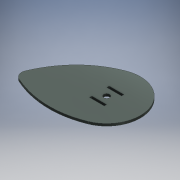
# Autodesk Inventor part: leva00
Saved by Autodesk Inventor 2016 (Build 200138000, 138)
## iProperties
Created: 2016-09-20
Part Number: leva00
Material: Madera (abedul)
Document SubType Name: Modeling
Designer: i95sa
Density: 0.55 g/cm^3
Appearance: Gris plomo - Pulido
Author: i95sa
Autodesk Inventor part; units mm, degrees
ref_plane "YZ Plane" through (0, 0, 0) normal (1, 0, 0) x (0, 1, 0)
ref_plane "XZ Plane" through (0, 0, 0) normal (0, 1, 0) x (-1, 0, 0)
ref_plane "XY Plane" through (0, 0, 0) normal (0, 0, 1) x (1, 0, 0)
sketch "Boceto1" plane through (0, 0, 0) normal (0, 0, 1) x (1, 0, 0)
  arc A0 (52.8206, 20.9132) -> (-52.8206, -20.9132) centre (0, 0) ccw
  arc A1 (-81.2867, -32.1837) -> (-105.6655, -41.8359) centre (-93.4761, -37.0098) ccw
  line L0 (-109.1946, -43.2332) -> (-114.0207, -31.0438)
  line L1 (-20.286, 53.0646) -> (-28.3295, 73.3802)
  line L2 (-28.3295, 73.3802) -> (-114.0207, -31.0438)
  line L3 (-114.0207, -31.0438) -> (-80.7549, 9.4942)
  arc A2 (-20.286, 53.0646) -> (-80.7549, 9.4942) centre (31.625, -82.7256) ccw
  arc A3 (-80.7549, 9.4942) -> (-105.5943, -32.0077) centre (46.1474, -94.6428) ccw
  line L4 (4.0631, 1.6087) -> (52.8206, 20.9132)
  line L5 (-4.0631, -1.6087) -> (-109.1946, -43.2332)
  arc A4 (-52.8206, -20.9132) -> (52.8206, 20.9132) centre (0, 0) ccw
  arc A5 (-105.6655, -41.8359) -> (-81.2867, -32.1837) centre (-93.4761, -37.0098) ccw
  line L6 (-109.1946, -43.2332) -> (-104.3685, -55.4226)
  line L7 (21.5374, -52.5692) -> (29.5809, -72.8848)
  line L8 (29.5809, -72.8848) -> (-104.3685, -55.4226)
  line L9 (-104.3685, -55.4226) -> (-52.3685, -62.2015)
  arc A6 (-52.3685, -62.2015) -> (21.5374, -52.5692) centre (-33.5759, 81.9532) ccw
  arc A7 (-98.8858, -48.9517) -> (-52.3685, -62.2015) centre (-31.1474, 100.5817) ccw
  dimension "d0" = 113.62
  dimension "d6" = 26.22
  dimension "d7" = 13.11
  dimension "d8" = 21.85
  dimension "d9" = 52.44
  constraints: 20 end point, 20 point on circle, 8 centre point, 6 symmetric about line, 5 point on line, 4 tangent, 1 collinear, 4 other
  measures "d0" diameter of A0
  measures "d6" diameter of A1
  measures "d7" distance of L0.start L0.end
  measures "d8" distance of L1.start L1.end
  measures "d9" distance of L0.end L3.end
extrude "Extrusión2" add sketch "Boceto1" along normal blind 4 contours A4 A0 | A0 L5 A1 A3 A2 | A6 A7 A5 L5 A4 | L5 A1 | A5 L5
sketch "Boceto2" plane through (0, 0, 4) normal (0, 0, 1) x (1, 0, 0)
  line L0 (0, 0) -> (0, 12.5)
  line L1 (0, 12.5) -> (-12.5, 12.5)
  line L2 (-12.5, 12.5) -> (-12.5, 16.7)
  line L3 (-12.5, 16.7) -> (12.5, 16.7)
  line L4 (12.5, 16.7) -> (12.5, 12.5)
  line L5 (12.5, 12.5) -> (0, 12.5)
  line L6 (0, 0) -> (12.5, 0)
  line L7 (0, 0) -> (0, -12.5)
  line L8 (0, -12.5) -> (-12.5, -12.5)
  line L9 (-12.5, -12.5) -> (-12.5, -16.7)
  line L10 (-12.5, -16.7) -> (12.5, -16.7)
  line L11 (12.5, -16.7) -> (12.5, -12.5)
  line L12 (12.5, -12.5) -> (0, -12.5)
  circle A0 centre (0, 0) radius 5
  dimension "d24" = 12.5
  dimension "d25" = 12.5
  dimension "d26" = 4.2
  dimension "d27" = 25
  dimension "d28" = 10
  constraints: 26 end point, 5 perpendicular, 5 symmetric about line, 3 point on line, 1 centre point, 1 coincident, 1 parallel, 1 vertical
  measures "d24" distance of L0.start L0.end
  measures "d25" distance of L0.end L1.end
  measures "d26" distance of L1.end L2.end
  measures "d27" distance of L2.end L3.end
  measures "d28" diameter of A0
extrude "Extrusión3" cut sketch "Boceto2" against normal blind 4
